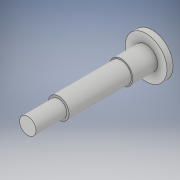
# Autodesk Inventor part: spindle
Saved by Autodesk Inventor 2018.3 (Build 223285000, 285)
## iProperties
Created: 2020-12-08
Part Number: spindle
Material: Generic
Document SubType Name: Modeling
Designer: Alex Dhawan
Density: 1 g/cm^3
Appearance: Default
Author: Alex Dhawan
Autodesk Inventor part; units mm, degrees
ref_plane "YZ Plane" through (0, 0, 0) normal (1, 0, 0) x (0, 1, 0)
ref_plane "XZ Plane" through (0, 0, 0) normal (0, 1, 0) x (-1, 0, 0)
ref_plane "XY Plane" through (0, 0, 0) normal (0, 0, 1) x (1, 0, 0)
sketch "Sketch1" plane through (0, 0, 0) normal (0, 0, 1) x (1, 0, 0)
  circle A0 centre (0, 0) radius 8.5
  dimension "d0" = 17
  constraints: 1 centre point, 1 coincident
  measures "d0" diameter of A0
extrude "Extrusion1" add sketch "Sketch1" against normal blind 51.2
sketch "Sketch2" plane through (0, 0, 0) normal (0, 0, 1) x (1, 0, 0)
  circle A0 centre (0, 0) radius 6.75
  dimension "d3" = 13.5
  constraints: 1 centre point, 1 coincident
  measures "d3" diameter of A0
extrude "Extrusion2" add sketch "Sketch2" along normal blind 25.3
sketch "Sketch3" plane through (0, 0, -51.2) normal (0, 0, -1) x (-1, 0, 0)
  circle A0 centre (0, 0) radius 9.5
  dimension "d6" = 19
  constraints: 1 centre point, 1 coincident
  measures "d6" diameter of A0
extrude "Extrusion3" add sketch "Sketch3" along normal blind 20.4952
sketch "Sketch4" plane through (0, 0, -71.6952) normal (0, 0, -1) x (-1, 0, 0)
  circle A0 centre (0, 0) radius 17.15
  dimension "d9" = 34.3
  constraints: 1 centre point, 1 coincident
  measures "d9" diameter of A0
extrude "Extrusion4" add sketch "Sketch4" along normal blind 5
body "Solid1"
